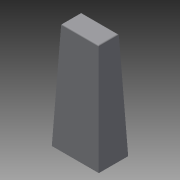
# Autodesk Inventor part: Foot
Saved by Autodesk Inventor 2015 (Build 190159000, 159)
## iProperties
Created: 2016-03-27
Part Number: Foot
Material: Generic
Document SubType Name: Modeling
Designer: Noah
Density: 1 g/cm^3
Appearance: Default
Author: Noah
Autodesk Inventor part; units mm, degrees
ref_plane "YZ Plane" through (0, 0, 0) normal (1, 0, 0) x (0, 1, 0)
ref_plane "XZ Plane" through (0, 0, 0) normal (0, 1, 0) x (-1, 0, 0)
ref_plane "XY Plane" through (0, 0, 0) normal (0, 0, 1) x (1, 0, 0)
sketch "Sketch1" plane through (0, 0, 0) normal (0, 0, 1) x (1, 0, 0)
  line L0 (-20, 12.5) -> (20, 12.5)
  line L1 (20, 12.5) -> (20, -12.5)
  line L2 (20, -12.5) -> (-20, -12.5)
  line L3 (-20, -12.5) -> (-20, 12.5)
  point P0 (0, 0)
  dimension "d0" = 40
  dimension "d1" = 25
  dimension "d2" = 12.5
  dimension "d3" = 20
  constraints: 8 end point, 2 parallel, 1 horizontal, 1 perpendicular
  measures "d0" distance of L1.end L2.end
  measures "d1" distance of L0.end L1.end
  measures "d2" distance from line of L0 point (0, 0)
  measures "d3" distance from line of L1 point (0, 0)
extrude "Extrusion1" add sketch "Sketch1" along normal blind 90
chamfer "Chamfer1" distance 4 distance2 90 1 edges at (0, 12.5, 90) measured on face at (-6.6667, 4.1667, 90)
chamfer "Chamfer2" distance 4 distance2 90 1 edges at (0, -12.5, 90) measured on face at (-6.6667, 1.5003, 90)
chamfer "Chamfer3" distance 4 distance2 90 1 edges at (20, 0, 90) measured on face at (-6.6667, 2.8335, 90)
chamfer "Chamfer4" distance 4 distance2 90 1 edges at (-20, 0, 90) measured on face at (-7.9998, 2.8335, 90)
fillet "Fillet1" radius 1 4 edges at (0, 8.5005, 90) (-16.0005, 0, 90) (0, -8.5005, 90) (16.0005, 0, 90)
body "Solid1"
